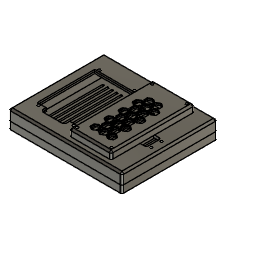
orient-beetle-screen-case-v2 v14 (Autodesk Fusion 360 design; units mm, degrees)
Autodesk Fusion 360 part; units mm, degrees
sketch "base-sketch" plane through (0, 0, 0) normal (0, 0, 1) x (1, 0, 0)
  line L0 (0, 0) -> (120, 0)
  line L1 (120, 0) -> (120, 100)
  line L2 (120, 100) -> (0, 100)
  line L3 (0, 100) -> (0, 0)
  line L4 (10, 19.5) -> (53.5, 19.5)
  line L5 (53.5, 19.5) -> (53.5, 80.5)
  line L6 (53.5, 80.5) -> (10, 80.5)
  line L7 (10, 80.5) -> (10, 19.5)
  line L8 (104, 11) -> (64, 11)
  line L9 (64, 11) -> (64, 89)
  line L10 (64, 89) -> (104, 89)
  line L11 (104, 89) -> (104, 11)
  line L12 (44.25, 86.5) -> (19.25, 86.5)
  line L13 (19.25, 86.5) -> (19.25, 80.5)
  line L14 (19.25, 80.5) -> (44.25, 80.5)
  line L15 (44.25, 80.5) -> (44.25, 86.5)
  line L16 (31.75, 19.5) -> (31.75, 80.5) construction
  line L17 (31.75, 80.5) -> (31.75, 86.5) construction
  line L18 (104, 49) -> (113.5, 49)
  line L19 (113.5, 49) -> (113.5, 65.5)
  line L20 (113.5, 65.5) -> (104, 65.5)
  line L21 (104, 65.5) -> (104, 49)
  circle A0 centre (116, 51.5) radius 1.5
  circle A1 centre (116, 63) radius 1.5
  line L22 (116, 51.5) -> (116, 63) construction
  line L23 (104, 57.25) -> (113.5, 57.25)
  circle A2 centre (12.25, 16.5) radius 1.6
  line L24 (10, 50) -> (53.5, 50) construction
  circle A3 centre (51.25, 16.5) radius 1.6
  circle A4 centre (12.25, 83.5) radius 1.6
  circle A5 centre (51.25, 83.5) radius 1.6
  line L25 (122.1, 102.1) -> (-2.1, 102.1)
  line L26 (-2.1, 102.1) -> (-2.1, -2.1)
  line L27 (-2.1, -2.1) -> (122.1, -2.1)
  line L28 (122.1, -2.1) -> (122.1, 102.1)
  point P0 (116, 57.25)
  dimension "d1" = 120
  dimension "d2" = 100
  dimension "d3" = 43.5
  dimension "d4" = 61
  dimension "d6" = 10
  dimension "d7" = 40
  dimension "d8" = 78
  dimension "d9" = 16
  dimension "d10" = 11
  dimension "d11" = 19.5
  dimension "d12" = 19.5
  dimension "d13" = 11
  dimension "d14" = 25
  dimension "d15" = 6
  dimension "d20" = 9.5
  dimension "d21" = 16.5
  dimension "d22" = 34.5
  dimension "d23" = 3
  dimension "d24" = 3
  dimension "d25" = 11.5
  dimension "d27" = 12
  dimension "d28" = 3.2
  dimension "d31" = 3.2
  dimension "d33" = 3.2
  dimension "d40" = 19.5
  dimension "d41" = 33.5
  dimension "d42" = 3.2
  dimension "d43" = 39
  dimension "d44" = 33.5
  dimension "d45" = 33.5
  dimension "d46" = 33.5
  dimension "d47" = 39
  dimension "d48" = 19.5
  dimension "d49" = 2.1
  constraint horizontal L0
  constraint vertical L1
  constraint horizontal L2
  constraint vertical L3
  constraint coincident L0.start L3.end
  constraint horizontal L4
  constraint vertical L5
  constraint horizontal L6
  constraint vertical L7
  constraint horizontal L8
  constraint vertical L9
  constraint horizontal L10
  constraint vertical L11
  constraint horizontal L12
  constraint vertical L13
  constraint horizontal L14
  constraint vertical L15
  constraint midpoint L4 L16.start
  constraint midpoint L6 L16.end
  constraint midpoint L14 L16.end
  constraint midpoint L12 L17.end
  constraint collinear L16 L17
  constraint collinear L6 L14
  constraint horizontal L18
  constraint vertical L19
  constraint horizontal L20
  constraint vertical L21
  constraint collinear L11 L21
  constraint coincident A0.centre L22.start
  constraint coincident A1.centre L22.end
  constraint parallel L19 L22
  constraint midpoint L21 L23.start
  constraint midpoint L19 L23.end
  constraint midpoint L22 P0
  constraint coincident L23 P0
  constraint midpoint L7 L24.start
  constraint midpoint L5 L24.end
  measures "d1" distance of L0.start L0.end
  measures "d2" distance of L0.start L2.end
  measures "d3" distance of L4.start L4.end
  measures "d4" distance of L4.start L6.end
  measures "d6" distance of L3 L7
  measures "d7" distance of L8.start L8.end
  measures "d8" distance of L8.start L10.end
  measures "d9" distance of L1 L11
  measures "d10" distance of L0 L8
  measures "d11" distance of L2 L6
  measures "d12" distance of L0 L4
  measures "d13" distance of L2 L10
  measures "d14" distance of L12.start L12.end
  measures "d15" distance of L12.end L13.end
  measures "d20" distance of L19.end L20.end
  measures "d21" distance of L18.end L19.end
  measures "d22" distance of L2 L20
  measures "d23" diameter of A0
  measures "d24" diameter of A1
  measures "d25" distance of A0.centre A1.centre
  measures "d27" distance of L21 A0.centre
  measures "d28" diameter of A2
  measures "d31" diameter of A3
  measures "d33" diameter of A4
  measures "d40" distance of L16 A4.centre
  measures "d41" distance of L24 A4.centre
  measures "d42" diameter of A5
  measures "d43" distance of A4.centre A5.centre
  measures "d44" distance of L24 A5.centre
  measures "d45" distance of A2.centre L24
  measures "d46" distance of L24 A3.centre
  measures "d47" distance of A2.centre A3.centre
  measures "d48" distance of L16 A2.centre
sketch "body-two-better" plane through (0, 0, 0) normal (0, 0, 1) x (1, 0, 0)
  line L0 (-14.1, 0) -> (-134.1, 0)
  line L1 (-134.1, 0) -> (-134.1, 100)
  line L2 (-134.1, 100) -> (-14.1, 100)
  line L3 (-14.1, 100) -> (-14.1, 0)
  line L4 (-2.1, 102.1) -> (-2.1, -2.1)
  line L5 (0, 0) -> (120, 0)
  line L6 (-11.6, -2.5) -> (-136.6, -2.5)
  line L7 (-136.6, -2.5) -> (-136.6, 102.5)
  line L8 (-136.6, 102.5) -> (-11.6, 102.5)
  line L9 (-11.6, 102.5) -> (-11.6, -2.5)
  line L10 (-103.1, 100) -> (-103.1, 0) construction
  line L11 (-14.1, 50) -> (-134.1, 50) construction
  line L12 (-81.35, 19.25) -> (-124.85, 19.25)
  line L13 (-124.85, 19.25) -> (-124.85, 80.75)
  line L14 (-124.85, 80.75) -> (-81.35, 80.75)
  line L15 (-81.35, 80.75) -> (-81.35, 19.25)
  line L16 (-103.1, 80.75) -> (-103.1, 19.25) construction
  line L17 (-81.35, 50) -> (-124.85, 50) construction
  circle A0 centre (-122.6, 83.5) radius 1.55
  circle A1 centre (-122.6, 16.5) radius 1.55
  line L18 (-122.6, 16.5) -> (-122.6, 26.5) construction
  line L19 (-122.6, 83.5) -> (-122.6, 73.5) construction
  circle A2 centre (-83.6, 83.5) radius 1.55
  line L20 (-83.6, 83.5) -> (-93.6, 83.5) construction
  line L21 (-122.6, 83.5) -> (-112.6, 83.5) construction
  circle A3 centre (-83.6, 16.5) radius 1.55
  line L22 (-83.6, 16.5) -> (-83.6, 26.5) construction
  line L23 (-83.6, 83.5) -> (-83.6, 73.5) construction
  line L24 (-83.6, 16.5) -> (-93.6, 16.5) construction
  line L25 (-122.6, 16.5) -> (-112.6, 16.5) construction
  line L26 (-83.6, 83.5) -> (-122.6, 16.5) construction
  line L27 (-117.1, 91.75) -> (-89.1, 91.75) construction
  line L28 (-89.1, 91.75) -> (-89.1, 80.75) construction
  line L29 (-89.1, 80.75) -> (-117.1, 80.75)
  line L30 (-117.1, 80.75) -> (-117.1, 91.75) construction
  line L31 (-117.1, 91.75) -> (-89.1, 80.75) construction
  line L32 (-89.1, 91.75) -> (-117.1, 80.75) construction
  line L33 (-53.1, 100) -> (-53.1, 0) construction
  line L34 (-73.1, 89) -> (-33.1, 89)
  line L35 (-33.1, 89) -> (-33.1, 11)
  line L36 (-33.1, 11) -> (-73.1, 11)
  line L37 (-73.1, 11) -> (-73.1, 89)
  line L38 (-73.1, 89) -> (-33.1, 11) construction
  line L39 (-33.1, 89) -> (-73.1, 11) construction
  line L40 (-33.1, 52) -> (-23.1, 52)
  line L41 (-23.1, 52) -> (-23.1, 36)
  line L42 (-23.1, 36) -> (-33.1, 36)
  line L43 (-33.1, 36) -> (-33.1, 52)
  line L44 (-33.1, 52) -> (-23.1, 36) construction
  line L45 (-23.1, 52) -> (-33.1, 36) construction
  circle A4 centre (-20.1, 49.75) radius 1.3
  circle A5 centre (-20.1, 38.25) radius 1.3
  line L46 (-20.1, 38.25) -> (-20.1, 42.25) construction
  line L47 (-20.1, 49.75) -> (-20.1, 45.75) construction
  line L48 (-20.1, 49.75) -> (-20.1, 38.25) construction
  line L49 (-23.1, 44) -> (-20.1, 44) construction
  circle A6 centre (-34.1, 91.5) radius 1.4
  circle A7 centre (-34.1, 8.5) radius 1.4
  circle A8 centre (-72.1, 8.5) radius 1.4
  circle A9 centre (-72.1, 91.5) radius 1.4
  line L50 (-34.1, 91.5) -> (-36.1, 91.5) construction
  line L51 (-34.1, 8.5) -> (-36.1, 8.5) construction
  line L52 (-34.1, 8.5) -> (-34.1, 10.5) construction
  line L53 (-72.1, 8.5) -> (-72.1, 10.5) construction
  line L54 (-72.1, 8.5) -> (-70.1, 8.5) construction
  line L55 (-72.1, 91.5) -> (-72.1, 89.5) construction
  line L56 (-72.1, 91.5) -> (-70.1, 91.5) construction
  line L57 (-34.1, 91.5) -> (-34.1, 89.5) construction
  line L58 (-34.1, 91.5) -> (-72.1, 8.5) construction
  line L59 (-115.1, 19.25) -> (-91.1, 19.25)
  line L60 (-91.1, 19.25) -> (-91.1, 13.25)
  line L61 (-91.1, 13.25) -> (-115.1, 13.25)
  line L62 (-115.1, 13.25) -> (-115.1, 19.25)
  line L63 (-115.1, 19.25) -> (-91.1, 13.25) construction
  line L64 (-91.1, 19.25) -> (-115.1, 13.25) construction
  line L65 (-28.1, 94) -> (-28.1, 6) construction
  line L66 (-28.1, 6) -> (-78.1, 6) construction
  line L67 (-78.1, 6) -> (-78.1, 94) construction
  line L68 (-78.1, 94) -> (-28.1, 94) construction
  point P0 (-103.1, 50)
  point P1 (-103.1, 50)
  point P2 (-103.1, 50)
  point P3 (-103.1, 80.75)
  point P4 (-103.1, 86.25)
  point P5 (-103.1, 80.75)
  point P6 (-53.1, 50)
  point P7 (-53.1, 50)
  point P8 (-28.1, 44)
  point P9 (-33.1, 44)
  point P10 (-33.1, 44)
  point P11 (-53.1, 50)
  point P12 (-103.1, 19.25)
  point P13 (-103.1, 16.25)
  point P14 (-103.1, 19.25)
  dimension "d150" = 120
  dimension "d151" = 100
  dimension "d152" = 12
  dimension "d153" = -2.5
  dimension "d154" = 31
  dimension "d155" = 43.5
  dimension "d156" = 61.5
  dimension "d157" = 3.1
  dimension "d158" = 3.1
  dimension "d159" = 10
  dimension "d160" = 10
  dimension "d162" = 3.1
  dimension "d163" = 10
  dimension "d164" = 39
  dimension "d165" = 67
  dimension "d166" = 3.1
  dimension "d167" = 10
  dimension "d168" = 10
  dimension "d169" = 10
  dimension "d170" = 10
  dimension "d171" = 10
  dimension "d174" = 28
  dimension "d175" = 11
  dimension "d176" = 50
  dimension "d177" = 40
  dimension "d178" = 78
  dimension "d179" = 16
  dimension "d180" = 10
  dimension "d184" = 2.6
  dimension "d185" = 2.6
  dimension "d186" = 4
  dimension "d187" = 4
  dimension "d188" = 11.5
  dimension "d190" = 3
  dimension "d198" = 2.8
  dimension "d199" = 2.8
  dimension "d200" = 2.8
  dimension "d201" = 2.8
  dimension "d206" = 2
  dimension "d207" = 2
  dimension "d208" = 2
  dimension "d209" = 2
  dimension "d210" = 2
  dimension "d211" = 2
  dimension "d212" = 2
  dimension "d213" = 2
  dimension "d214" = 83
  dimension "d215" = 38
  dimension "d224" = 44
  dimension "d225" = 6
  dimension "d227" = 24
  dimension "d247" = -5
  constraint horizontal L0
  constraint vertical L1
  constraint horizontal L2
  constraint vertical L3
  constraint collinear L0 L5
  constraint coincident L2 L10.start
  constraint coincident L0 L10.end
  constraint perpendicular L0 L10
  constraint midpoint L3 L11.start
  constraint midpoint L1 L11.end
  constraint horizontal L12
  constraint vertical L13
  constraint horizontal L14
  constraint vertical L15
  constraint midpoint L10 P2
  constraint midpoint L14 P5
  constraint midpoint L12 P14
  constraint midpoint L15 L17.start
  constraint midpoint L13 L17.end
  constraint midpoint L17 P2
  constraint coincident A1.centre L18.start
  constraint vertical L18
  constraint coincident A0.centre L19.start
  constraint vertical L19
  constraint collinear L18 L19
  constraint coincident A2.centre L20.start
  constraint horizontal L20
  constraint perpendicular L19 L21
  constraint collinear L20 L21
  constraint coincident A3.centre L22.start
  constraint vertical L22
  constraint perpendicular L20 L23
  constraint collinear L22 L23
  constraint perpendicular L22 L24
  constraint perpendicular L18 L25
  constraint collinear L24 L25
  constraint midpoint L26 P2
  constraint midpoint L16 P2
  constraint coincident P5 P3
  constraint horizontal L27
  constraint perpendicular L27 L28
  constraint parallel L27 L29
  constraint parallel L28 L30
  constraint coincident L31 P4
  constraint coincident L32 P4
  constraint midpoint L29 P5
  constraint vertical L33
  constraint coincident L2 L33.start
  constraint coincident L0 L33.end
  constraint midpoint L33 P11
  constraint horizontal L34
  constraint perpendicular L34 L35
  constraint parallel L34 L36
  constraint parallel L35 L37
  constraint coincident L38 P11
  constraint coincident L39 P11
  constraint coincident P11 P7
  constraint horizontal L40
  constraint perpendicular L40 L41
  constraint parallel L40 L42
  constraint parallel L41 L43
  constraint coincident L44 P8
  constraint coincident L45 P8
  constraint coincident A5.centre L46.start
  constraint vertical L46
  constraint coincident A4.centre L47.start
  constraint vertical L47
  constraint collinear L46 L47
  constraint midpoint L41 L49.start
  constraint perpendicular L41 L49
  constraint midpoint L48 L49.end
  constraint coincident L35 P10
  constraint midpoint L43 P10
  constraint coincident P10 P9
  constraint coincident A6.centre L50.start
  constraint horizontal L50
  constraint coincident A7.centre L51.start
  constraint horizontal L51
  constraint perpendicular L51 L52
  constraint coincident A8.centre L53.start
  constraint vertical L53
  constraint perpendicular L53 L54
  constraint coincident A9.centre L55.start
  constraint vertical L55
  constraint perpendicular L55 L56
  constraint vertical L57
  constraint collinear L50 L56
  constraint collinear L53 L55
  constraint collinear L51 L54
  constraint collinear L52 L57
  constraint midpoint L58 P11
  constraint coincident P14 P12
  constraint horizontal L59
  constraint perpendicular L59 L60
  constraint parallel L59 L61
  constraint parallel L60 L62
  constraint coincident L63 P13
  constraint coincident L64 P13
  constraint midpoint L59 P14
  measures "d150" distance of L0.start L0.end
  measures "d151" distance of L0.start L2.end
  measures "d152" distance of L3 L4
  measures "d154" distance of L1 L10
  measures "d155" distance of L12.start L12.end
  measures "d156" distance of L12.start L14.end
  measures "d157" diameter of A0
  measures "d158" diameter of A1
  measures "d159" distance of A0.centre L19.end
  measures "d160" distance of A1.centre L18.end
  measures "d162" diameter of A2
  measures "d163" distance of A2.centre L20.end
  measures "d164" distance of A0.centre A2.centre
  measures "d165" distance of A0.centre A1.centre
  measures "d166" diameter of A3
  measures "d167" distance of A3.centre L22.end
  measures "d168" distance of A2.centre L23.end
  measures "d169" distance of A3.centre L24.end
  measures "d170" distance of A1.centre L25.end
  measures "d171" distance of A0.centre L21.end
  measures "d174" distance of L28.end L29.end
  measures "d175" distance of L27.end L28.end
  measures "d176" distance of L10 L33
  measures "d177" distance of L35.end L36.end
  measures "d178" distance of L34.start L36.end
  measures "d179" distance of L40.end L41.end
  measures "d180" distance of L40.start L40.end
  measures "d184" diameter of A4
  measures "d185" diameter of A5
  measures "d186" distance of A5.centre L46.end
  measures "d187" distance of A4.centre L47.end
  measures "d188" distance of A4.centre A5.centre
  measures "d190" distance of L49.start L49.end
  measures "d198" diameter of A6
  measures "d199" diameter of A7
  measures "d200" diameter of A8
  measures "d201" diameter of A9
  measures "d206" distance of A7.centre L51.end
  measures "d207" distance of A7.centre L52.end
  measures "d208" distance of A8.centre L53.end
  measures "d209" distance of A8.centre L54.end
  measures "d210" distance of A9.centre L55.end
  measures "d211" distance of A9.centre L56.end
  measures "d212" distance of A6.centre L57.end
  measures "d213" distance of A6.centre L50.end
  measures "d214" distance of A6.centre A7.centre
  measures "d215" distance of A7.centre A8.centre
  measures "d224" distance of L0 P8
  measures "d225" distance of L59.start L61.end
  measures "d227" distance of L60.end L61.end
extrude "wall-extrude" add sketch "body-two-better" against normal blind 10 contours L6 L7 L8 L9 makes body 1
extrude "face-extrude" add sketch "body-two-better" against normal blind 3 contours L0 L1 L2 L3 bodies 1
sketch "expansion-sketch" plane through (0, 0, 0) normal (0, 0, 1) x (1, 0, 0)
  line L0 (-78.1, 6) -> (-78.1, 94)
  line L1 (-78.1, 94) -> (-28.1, 94)
  line L2 (-28.1, 6) -> (-78.1, 6)
  line L3 (-28.1, 94) -> (-28.1, 6)
  line L4 (-53.1, 94) -> (-53.1, 6) construction
  line L5 (-78.1, 50) -> (-28.1, 50) construction
  line L6 (-53.1, 54) -> (-56.5641, 52)
  line L7 (-56.5641, 52) -> (-56.5641, 48)
  line L8 (-56.5641, 48) -> (-53.1, 46)
  line L9 (-53.1, 46) -> (-49.6359, 48)
  line L10 (-49.6359, 48) -> (-49.6359, 52)
  line L11 (-49.6359, 52) -> (-53.1, 54)
  line L12 (-44.1, 46) -> (-40.6359, 48)
  line L13 (-40.6359, 48) -> (-40.6359, 52)
  line L14 (-40.6359, 52) -> (-44.1, 54)
  line L15 (-44.1, 54) -> (-47.5641, 52)
  line L16 (-47.5641, 48) -> (-44.1, 46)
  line L17 (-47.5641, 52) -> (-47.5641, 48)
  line L18 (-62.1, 46) -> (-58.6359, 48)
  line L19 (-58.6359, 48) -> (-58.6359, 52)
  line L20 (-58.6359, 52) -> (-62.1, 54)
  line L21 (-62.1, 54) -> (-65.5641, 52)
  line L22 (-65.5641, 48) -> (-62.1, 46)
  line L23 (-65.5641, 52) -> (-65.5641, 48)
  line L24 (-53.1, 50) -> (-54.8321, 53) construction
  line L25 (-53.1, 50) -> (-51.3679, 53) construction
  line L26 (-48.6, 61.7942) -> (-52.0641, 59.7942)
  line L27 (-52.0641, 59.7942) -> (-52.0641, 55.7942)
  line L28 (-52.0641, 55.7942) -> (-48.6, 53.7942)
  line L29 (-48.6, 53.7942) -> (-45.1359, 55.7942)
  line L30 (-45.1359, 59.7942) -> (-48.6, 61.7942)
  line L31 (-45.1359, 55.7942) -> (-45.1359, 59.7942)
  line L32 (-57.6, 61.7942) -> (-61.0641, 59.7942)
  line L33 (-61.0641, 59.7942) -> (-61.0641, 55.7942)
  line L34 (-61.0641, 55.7942) -> (-57.6, 53.7942)
  line L35 (-57.6, 53.7942) -> (-54.1359, 55.7942)
  line L36 (-54.1359, 59.7942) -> (-57.6, 61.7942)
  line L37 (-54.1359, 55.7942) -> (-54.1359, 59.7942)
  line L38 (-62.1, 69.5) -> (-65.5641, 67.5)
  line L39 (-65.5641, 67.5) -> (-65.5641, 63.5)
  line L40 (-65.5641, 63.5) -> (-62.1, 61.5)
  line L41 (-62.1, 61.5) -> (-58.6359, 63.5)
  line L42 (-58.6359, 67.5) -> (-62.1, 69.5)
  line L43 (-58.6359, 63.5) -> (-58.6359, 67.5)
  line L44 (-54.1359, 75.2942) -> (-57.6, 77.2942)
  line L45 (-57.6, 77.2942) -> (-61.0641, 75.2942)
  line L46 (-61.0641, 75.2942) -> (-61.0641, 71.2942)
  line L47 (-61.0641, 71.2942) -> (-57.6, 69.2942)
  line L48 (-54.1359, 71.2942) -> (-54.1359, 75.2942)
  line L49 (-57.6, 69.2942) -> (-54.1359, 71.2942)
  line L50 (-48.6, 69.2942) -> (-45.1359, 71.2942)
  line L51 (-45.1359, 71.2942) -> (-45.1359, 75.2942)
  line L52 (-45.1359, 75.2942) -> (-48.6, 77.2942)
  line L53 (-48.6, 77.2942) -> (-52.0641, 75.2942)
  line L54 (-52.0641, 71.2942) -> (-48.6, 69.2942)
  line L55 (-52.0641, 75.2942) -> (-52.0641, 71.2942)
  line L56 (-53.1, 69.5) -> (-56.5641, 67.5)
  line L57 (-56.5641, 67.5) -> (-56.5641, 63.5)
  line L58 (-56.5641, 63.5) -> (-53.1, 61.5)
  line L59 (-53.1, 61.5) -> (-49.6359, 63.5)
  line L60 (-49.6359, 67.5) -> (-53.1, 69.5)
  line L61 (-49.6359, 63.5) -> (-49.6359, 67.5)
  line L62 (-40.6359, 67.5) -> (-44.1, 69.5)
  line L63 (-44.1, 69.5) -> (-47.5641, 67.5)
  line L64 (-47.5641, 67.5) -> (-47.5641, 63.5)
  line L65 (-47.5641, 63.5) -> (-44.1, 61.5)
  line L66 (-40.6359, 63.5) -> (-40.6359, 67.5)
  line L67 (-44.1, 61.5) -> (-40.6359, 63.5)
  line L68 (-62.1, 38.5) -> (-65.5641, 36.5)
  line L69 (-65.5641, 36.5) -> (-65.5641, 32.5)
  line L70 (-65.5641, 32.5) -> (-62.1, 30.5)
  line L71 (-62.1, 30.5) -> (-58.6359, 32.5)
  line L72 (-58.6359, 36.5) -> (-62.1, 38.5)
  line L73 (-58.6359, 32.5) -> (-58.6359, 36.5)
  line L74 (-54.1359, 44.2942) -> (-57.6, 46.2942)
  line L75 (-57.6, 46.2942) -> (-61.0641, 44.2942)
  line L76 (-61.0641, 44.2942) -> (-61.0641, 40.2942)
  line L77 (-61.0641, 40.2942) -> (-57.6, 38.2942)
  line L78 (-54.1359, 40.2942) -> (-54.1359, 44.2942)
  line L79 (-57.6, 38.2942) -> (-54.1359, 40.2942)
  line L80 (-48.6, 38.2942) -> (-45.1359, 40.2942)
  line L81 (-45.1359, 40.2942) -> (-45.1359, 44.2942)
  line L82 (-45.1359, 44.2942) -> (-48.6, 46.2942)
  line L83 (-48.6, 46.2942) -> (-52.0641, 44.2942)
  line L84 (-52.0641, 40.2942) -> (-48.6, 38.2942)
  line L85 (-52.0641, 44.2942) -> (-52.0641, 40.2942)
  line L86 (-53.1, 38.5) -> (-56.5641, 36.5)
  line L87 (-56.5641, 36.5) -> (-56.5641, 32.5)
  line L88 (-56.5641, 32.5) -> (-53.1, 30.5)
  line L89 (-53.1, 30.5) -> (-49.6359, 32.5)
  line L90 (-49.6359, 36.5) -> (-53.1, 38.5)
  line L91 (-49.6359, 32.5) -> (-49.6359, 36.5)
  line L92 (-40.6359, 36.5) -> (-44.1, 38.5)
  line L93 (-44.1, 38.5) -> (-47.5641, 36.5)
  line L94 (-47.5641, 36.5) -> (-47.5641, 32.5)
  line L95 (-47.5641, 32.5) -> (-44.1, 30.5)
  line L96 (-40.6359, 32.5) -> (-40.6359, 36.5)
  line L97 (-44.1, 30.5) -> (-40.6359, 32.5)
  line L98 (-62.1, 23) -> (-65.5641, 21)
  line L99 (-65.5641, 21) -> (-65.5641, 17)
  line L100 (-65.5641, 17) -> (-62.1, 15)
  line L101 (-62.1, 15) -> (-58.6359, 17)
  line L102 (-58.6359, 21) -> (-62.1, 23)
  line L103 (-58.6359, 17) -> (-58.6359, 21)
  line L104 (-54.1359, 28.7942) -> (-57.6, 30.7942)
  line L105 (-57.6, 30.7942) -> (-61.0641, 28.7942)
  line L106 (-61.0641, 28.7942) -> (-61.0641, 24.7942)
  line L107 (-61.0641, 24.7942) -> (-57.6, 22.7942)
  line L108 (-54.1359, 24.7942) -> (-54.1359, 28.7942)
  line L109 (-57.6, 22.7942) -> (-54.1359, 24.7942)
  line L110 (-48.6, 22.7942) -> (-45.1359, 24.7942)
  line L111 (-45.1359, 24.7942) -> (-45.1359, 28.7942)
  line L112 (-45.1359, 28.7942) -> (-48.6, 30.7942)
  line L113 (-48.6, 30.7942) -> (-52.0641, 28.7942)
  line L114 (-52.0641, 24.7942) -> (-48.6, 22.7942)
  line L115 (-52.0641, 28.7942) -> (-52.0641, 24.7942)
  line L116 (-53.1, 23) -> (-56.5641, 21)
  line L117 (-56.5641, 21) -> (-56.5641, 17)
  line L118 (-56.5641, 17) -> (-53.1, 15)
  line L119 (-53.1, 15) -> (-49.6359, 17)
  line L120 (-49.6359, 21) -> (-53.1, 23)
  line L121 (-49.6359, 17) -> (-49.6359, 21)
  line L122 (-40.6359, 21) -> (-44.1, 23)
  line L123 (-44.1, 23) -> (-47.5641, 21)
  line L124 (-47.5641, 21) -> (-47.5641, 17)
  line L125 (-47.5641, 17) -> (-44.1, 15)
  line L126 (-40.6359, 17) -> (-40.6359, 21)
  line L127 (-44.1, 15) -> (-40.6359, 17)
  point P0 (-53.1, 50)
  point P1 (-53.1, 50)
  dimension "d266" = 4
  dimension "d267" = 60
  dimension "d270" = 9
  dimension "d271" = 0
  dimension "d278" = 9
  dimension "d279" = 9
  dimension "d282" = 15.5
  dimension "d283" = 0
  constraint midpoint L1 L4.start
  constraint midpoint L2 L4.end
  constraint midpoint L0 L5.start
  constraint midpoint L3 L5.end
  constraint midpoint L5 P1
  constraint coincident P1 P0
  constraint midpoint L6 L24.end
  constraint midpoint L11 L25.end
  measures "d266" distance of L6.start P1
  measures "d267" angle of L3 L11
extrude "expansion-extrude" add sketch "expansion-sketch" along normal blind 8 separate body makes body 2
extrude "expansion-extrude-cut" cut sketch "body-two-better" along normal blind 6 contours L34 L35 L36 L37 L43 bodies 1 2
extrude "Extrude20" cut sketch "body-two-better" along normal blind 20 contours A6 | A7 | A8 | A9 bodies 2
move_face "OffsetFaces5" offset -2 2 faces at (-78.1, 35.3333, 2.6667) (-28.1, 64.6667, 2.6667) on bodies 2
move_face "OffsetFaces6" offset 2 2 faces at (-45.4333, 6, 2.6667) (-60.7667, 94, 2.6667) on bodies 2
sketch "cable-cut" plane through (0, 102.5, 0) normal (0, 1, 0) x (-1, 0, 0)
  line L0 (136.6, 0) -> (11.6, 0)
  line L1 (11.6, -10) -> (136.6, -10)
  line L2 (65.1, 6) -> (41.1, 6)
  line L3 (41.1, 6) -> (41.1, -7)
  line L4 (41.1, -7) -> (65.1, -7)
  line L5 (65.1, -7) -> (65.1, 6)
  line L6 (65.1, 6) -> (41.1, -7) construction
  line L7 (41.1, 6) -> (65.1, -7) construction
  line L8 (76.1, 4) -> (30.1, 4) construction
  line L9 (65.1, 4) -> (41.1, 4) construction
  line L10 (11.6, 0) -> (11.6, -10)
  line L11 (136.6, -10) -> (136.6, 0)
  line L12 (76.1, 0) -> (76.1, 8)
  line L13 (30.1, 0) -> (30.1, 8)
  point P0 (53.1, -0.5)
  point P1 (53.1, 4)
  point P2 (53.1, 4)
  dimension "d294" = 24
  dimension "d295" = 13
  dimension "d296" = 2
  constraint horizontal L2
  constraint perpendicular L2 L3
  constraint parallel L2 L4
  constraint parallel L3 L5
  constraint coincident L6 P0
  constraint coincident L7 P0
  constraint midpoint L8 P2
  constraint coincident L5 L9.start
  constraint coincident L3 L9.end
  constraint perpendicular L3 L9
  constraint midpoint L9 P2
  constraint coincident P2 P1
  constraint midpoint L8.start L12
  constraint midpoint L8.end L13
  measures "d294" distance of L3.end L4.end
  measures "d295" distance of L2.end L3.end
  measures "d296" distance of L2 L9
extrude "Extrude21" cut sketch "cable-cut" against normal blind 39 contours L0 L3 L4 L5 bodies 1
extrude "Extrude22" cut sketch "cable-cut" against normal blind 40 contours L0 L2 L3 L5 bodies 2
extrude "Extrude23" add 1 faces at (-54.1, -1.6667, -10) along direction (0, 0, -1) blind 10 on bodies 1 bodies 1
sketch "bottom-sketch" plane through (0, 0, -20) normal (0, 0, -1) x (1, 0, 0)
  line L0 (-14.1, -100) -> (-134.1, -100)
  line L1 (-134.1, -100) -> (-134.1, 0)
  line L2 (-134.1, 0) -> (-14.1, 0)
  line L3 (-14.1, 0) -> (-14.1, -100)
  line L4 (-136.6, -102.5) -> (-11.6, -102.5)
  line L5 (-11.6, -102.5) -> (-11.6, 2.5)
  line L6 (-11.6, 2.5) -> (-136.6, 2.5)
  line L7 (-136.6, 2.5) -> (-136.6, -102.5)
  line L8 (-14.1, 0) -> (-134.1, 0)
  line L9 (-14.1, -100) -> (-14.1, 0)
  line L10 (-134.1, -100) -> (-14.1, -100)
  line L11 (-134.1, 0) -> (-134.1, -100)
extrude "Extrude24" add sketch "bottom-sketch" against normal blind 2 contours L0 L1 L2 L3 L8 L9 L10 L11 bodies 1
ref_plane "WorkPlane1" through (0, 0, -12) normal (0, 0, 1) x (1, 0, 0)
split "Split1" by plane through (0, 0, -12) normal (0, 0, 1) bodies 1 makes body 3 at (-21.4463, 80.8218, 0)
sketch "inner-sketch" plane through (0, 0, -18) normal (0, 0, 1) x (-1, 0, 0)
  line L0 (134.1, -100) -> (134.1, 0)
  line L1 (134.1, 0) -> (14.1, 0)
  line L2 (14.1, 0) -> (14.1, -100)
  line L3 (14.1, -100) -> (134.1, -100)
  line L4 (132.1, -98) -> (132.1, -2)
  line L5 (132.1, -2) -> (16.1, -2)
  line L6 (16.1, -2) -> (16.1, -98)
  line L7 (16.1, -98) -> (132.1, -98)
  dimension "d312" = -2
extrude "Extrude25" add sketch "inner-sketch" along normal blind 8 bodies 1
fillet "Fillet29" radius 2 8 edges at (-76.1, 4, 4) (-30.1, 4, 4) (-33.1, 89, 3) (-30.1, 96, 4) (-73.1, 89, 3) (-76.1, 96, 4) (-73.1, 11, 3) (-33.1, 11, 3) on bodies 2
fillet "Fillet30" radius 2 2 edges at (-41.1, 92.5, 6) (-65.1, 92.5, 6) on bodies 2
fillet "Fillet32" radius 2 23 edges at (-11.6, -2.5, -6) (-136.6, -2.5, -6) (-136.6, 102.5, -6) (-11.6, 102.5, -6) (-14.1, 100, -7.5) (-14.1, 0, -7.5) (-134.1, 0, -7.5) (-134.1, 100, -7.5) (-65.1, 89, -1.5) (-41.1, 89, -1.5) (-23.1, 36, -1.5) (-33.1, 36, -1.5) (-33.1, 52, -1.5) (-33.1, 11, -1.5) (-73.1, 11, -1.5) (-73.1, 89, -1.5) (-23.1, 52, -1.5) (-65.1, 101.25, -7) (-41.1, 101.25, -7) (-91.1, 13.25, -1.5) (-115.1, 13.25, -1.5) (-115.1, 19.25, -1.5) (-91.1, 19.25, -1.5) on bodies 3
chamfer "Chamfer1" distance 1 angle 45 12 edges at (-124.85, 50, 0) (-103.1, 80.75, 0) (-81.35, 50, 0) (-85.225, 19.25, 0) (-90.5142, 18.6642, 0) (-91.1, 16.25, 0) (-91.6858, 13.8358, 0) (-103.1, 13.25, 0) (-114.5142, 13.8358, 0) (-115.1, 16.25, 0) (-115.6858, 18.6642, 0) (-120.975, 19.25, 0) on bodies 3
chamfer "Chamfer2" distance 2 angle 45 9 edges at (-136.6, 50, 0) (-136.0142, -1.9142, 0) (-74.1, -2.5, 0) (-12.1858, -1.9142, 0) (-11.6, 50, 0) (-12.1858, 101.9142, 0) (-27.35, 102.5, 0) (-99.85, 102.5, 0) (-136.0142, 101.9142, 0) on bodies 3
chamfer "Chamfer3" distance 2 angle 45 8 edges at (-53.1, 96, 8) (-75.5142, 95.4142, 8) (-76.1, 50, 8) (-75.5142, 4.5858, 8) (-53.1, 4, 8) (-30.6858, 4.5858, 8) (-30.1, 50, 8) (-30.6858, 95.4142, 8) on bodies 2
chamfer "Chamfer4" distance 0.5 angle 45 120 edges at (-47.5641, 34.5, 8) (-45.8321, 31.5, 8) (-42.3679, 31.5, 8) (-42.3679, 37.5, 8) (-45.8321, 37.5, 8) (-40.6359, 34.5, 8) (-49.6359, 34.5, 8) (-51.3679, 31.5, 8) (-54.8321, 31.5, 8) (-56.5641, 34.5, 8) (-54.8321, 37.5, 8) (-51.3679, 37.5, 8) (-60.3679, 37.5, 8) (-63.8321, 37.5, 8) (-65.5641, 34.5, 8) (-63.8321, 31.5, 8) (-60.3679, 31.5, 8) (-58.6359, 34.5, 8) (-61.0641, 26.7942, 8) (-59.3321, 29.7942, 8) (-55.8679, 29.7942, 8) (-54.1359, 26.7942, 8) (-55.8679, 23.7942, 8) (-59.3321, 23.7942, 8) (-52.0641, 26.7942, 8) (-50.3321, 29.7942, 8) (-46.8679, 29.7942, 8) (-45.1359, 26.7942, 8) (-46.8679, 23.7942, 8) (-50.3321, 23.7942, 8) (-51.3679, 22, 8) (-54.8321, 22, 8) (-56.5641, 19, 8) (-54.8321, 16, 8) (-51.3679, 16, 8) (-49.6359, 19, 8) (-47.5641, 19, 8) (-45.8321, 16, 8) (-42.3679, 16, 8) (-40.6359, 19, 8) (-42.3679, 22, 8) (-45.8321, 22, 8) (-58.6359, 19, 8) (-60.3679, 16, 8) (-63.8321, 16, 8) (-65.5641, 19, 8) (-63.8321, 22, 8) (-60.3679, 22, 8) (-61.0641, 42.2942, 8) (-59.3321, 39.2942, 8) (-55.8679, 39.2942, 8) (-54.1359, 42.2942, 8) (-55.8679, 45.2942, 8) (-59.3321, 45.2942, 8) (-52.0641, 42.2942, 8) (-50.3321, 39.2942, 8) (-46.8679, 39.2942, 8) (-45.1359, 42.2942, 8) (-46.8679, 45.2942, 8) (-50.3321, 45.2942, 8) (-61.0641, 57.7942, 8) (-59.3321, 54.7942, 8) (-55.8679, 54.7942, 8) (-54.1359, 57.7942, 8) (-59.3321, 60.7942, 8) (-55.8679, 60.7942, 8) (-65.5641, 50, 8) (-63.8321, 47, 8) (-60.3679, 47, 8) (-63.8321, 53, 8) (-60.3679, 53, 8) (-58.6359, 50, 8) (-56.5641, 50, 8) (-54.8321, 47, 8) (-51.3679, 47, 8) (-49.6359, 50, 8) (-51.3679, 53, 8) (-54.8321, 53, 8) (-45.8321, 53, 8) (-47.5641, 50, 8) (-45.8321, 47, 8) (-42.3679, 47, 8) (-40.6359, 50, 8) (-42.3679, 53, 8) (-46.8679, 54.7942, 8) (-50.3321, 54.7942, 8) (-52.0641, 57.7942, 8) (-50.3321, 60.7942, 8) (-46.8679, 60.7942, 8) (-45.1359, 57.7942, 8) (-40.6359, 65.5, 8) (-42.3679, 68.5, 8) (-45.8321, 68.5, 8) (-47.5641, 65.5, 8) (-45.8321, 62.5, 8) (-42.3679, 62.5, 8) (-51.3679, 62.5, 8) (-58.6359, 65.5, 8) (-54.8321, 62.5, 8) (-56.5641, 65.5, 8) (-54.8321, 68.5, 8) (-51.3679, 68.5, 8) (-49.6359, 65.5, 8) (-60.3679, 68.5, 8) (-63.8321, 68.5, 8) (-65.5641, 65.5, 8) (-63.8321, 62.5, 8) (-60.3679, 62.5, 8) (-59.3321, 70.2942, 8) (-61.0641, 73.2942, 8) (-59.3321, 76.2942, 8) (-55.8679, 76.2942, 8) (-54.1359, 73.2942, 8) (-55.8679, 70.2942, 8) (-52.0641, 73.2942, 8) (-50.3321, 76.2942, 8) (-46.8679, 76.2942, 8) (-45.1359, 73.2942, 8) (-46.8679, 70.2942, 8) (-50.3321, 70.2942, 8) on bodies 2
move_face "OffsetFaces7" offset -0.5 4 faces at (-14.1, 33.3333, -11.3333) (-54.1, 0, -10.6667) (-134.1, 66.6667, -11.3333) (-54.1, 100, -11.3333) on bodies 1
fillet "Fillet33" radius 2 12 edges at (-11.6, 102.5, -16) (-14.6, 99.5, -11) (-11.6, -2.5, -16) (-14.6, 0.5, -11) (-136.6, -2.5, -16) (-133.6, 0.5, -11) (-136.6, 102.5, -16) (-133.6, 99.5, -11) (-16.1, 98, -14) (-132.1, 98, -14) (-132.1, 2, -14) (-16.1, 2, -14) on bodies 1
sketch "bottom-cut-sketch" plane through (0, 0, -20) normal (0, 0, -1) x (1, 0, 0)
  arc A0 (-136.6, -100.5) -> (-134.6, -102.5) centre (-134.6, -100.5) ccw
  line L0 (-134.6, -102.5) -> (-13.6, -102.5)
  arc A1 (-13.6, -102.5) -> (-11.6, -100.5) centre (-13.6, -100.5) ccw
  line L1 (-11.6, -100.5) -> (-11.6, 0.5)
  arc A2 (-11.6, 0.5) -> (-13.6, 2.5) centre (-13.6, 0.5) ccw
  line L2 (-13.6, 2.5) -> (-134.6, 2.5)
  arc A3 (-134.6, 2.5) -> (-136.6, 0.5) centre (-134.6, 0.5) ccw
  line L3 (-136.6, 0.5) -> (-136.6, -100.5)
  line L4 (-132.1, -98) -> (-132.1, -2)
  line L5 (-132.1, -2) -> (-16.1, -2)
  line L6 (-16.1, -2) -> (-16.1, -98)
  line L7 (-16.1, -98) -> (-132.1, -98)
  line L8 (-74.1, -2) -> (-74.1, -98) construction
  line L9 (-73.1, -10) -> (-75.1, -10)
  line L10 (-75.1, -10) -> (-75.1, -90)
  line L11 (-75.1, -90) -> (-73.1, -90)
  line L12 (-73.1, -90) -> (-73.1, -10)
  line L13 (-73.1, -10) -> (-75.1, -90) construction
  line L14 (-75.1, -10) -> (-73.1, -90) construction
  line L15 (-30.1, -10) -> (-30.1, -90)
  line L16 (-30.1, -90) -> (-28.1, -90)
  line L17 (-28.1, -10) -> (-30.1, -10)
  line L18 (-28.1, -90) -> (-28.1, -10)
  line L19 (-35.1, -10) -> (-35.1, -90)
  line L20 (-35.1, -90) -> (-33.1, -90)
  line L21 (-33.1, -10) -> (-35.1, -10)
  line L22 (-33.1, -90) -> (-33.1, -10)
  line L23 (-40.1, -10) -> (-40.1, -90)
  line L24 (-40.1, -90) -> (-38.1, -90)
  line L25 (-38.1, -10) -> (-40.1, -10)
  line L26 (-38.1, -90) -> (-38.1, -10)
  line L27 (-45.1, -10) -> (-45.1, -90)
  line L28 (-45.1, -90) -> (-43.1, -90)
  line L29 (-43.1, -10) -> (-45.1, -10)
  line L30 (-43.1, -90) -> (-43.1, -10)
  line L31 (-50.1, -10) -> (-50.1, -90)
  line L32 (-50.1, -90) -> (-48.1, -90)
  line L33 (-48.1, -10) -> (-50.1, -10)
  line L34 (-48.1, -90) -> (-48.1, -10)
  line L35 (-55.1, -10) -> (-55.1, -90)
  line L36 (-55.1, -90) -> (-53.1, -90)
  line L37 (-53.1, -10) -> (-55.1, -10)
  line L38 (-53.1, -90) -> (-53.1, -10)
  line L39 (-60.1, -10) -> (-60.1, -90)
  line L40 (-60.1, -90) -> (-58.1, -90)
  line L41 (-58.1, -10) -> (-60.1, -10)
  line L42 (-58.1, -90) -> (-58.1, -10)
  line L43 (-65.1, -10) -> (-65.1, -90)
  line L44 (-65.1, -90) -> (-63.1, -90)
  line L45 (-63.1, -10) -> (-65.1, -10)
  line L46 (-63.1, -90) -> (-63.1, -10)
  line L47 (-70.1, -10) -> (-70.1, -90)
  line L48 (-70.1, -90) -> (-68.1, -90)
  line L49 (-68.1, -10) -> (-70.1, -10)
  line L50 (-68.1, -90) -> (-68.1, -10)
  line L51 (-80.1, -10) -> (-80.1, -90)
  line L52 (-80.1, -90) -> (-78.1, -90)
  line L53 (-78.1, -10) -> (-80.1, -10)
  line L54 (-78.1, -90) -> (-78.1, -10)
  line L55 (-85.1, -10) -> (-85.1, -90)
  line L56 (-85.1, -90) -> (-83.1, -90)
  line L57 (-83.1, -10) -> (-85.1, -10)
  line L58 (-83.1, -90) -> (-83.1, -10)
  line L59 (-90.1, -10) -> (-90.1, -90)
  line L60 (-90.1, -90) -> (-88.1, -90)
  line L61 (-88.1, -10) -> (-90.1, -10)
  line L62 (-88.1, -90) -> (-88.1, -10)
  line L63 (-95.1, -10) -> (-95.1, -90)
  line L64 (-95.1, -90) -> (-93.1, -90)
  line L65 (-93.1, -10) -> (-95.1, -10)
  line L66 (-93.1, -90) -> (-93.1, -10)
  line L67 (-100.1, -10) -> (-100.1, -90)
  line L68 (-100.1, -90) -> (-98.1, -90)
  line L69 (-98.1, -10) -> (-100.1, -10)
  line L70 (-98.1, -90) -> (-98.1, -10)
  line L71 (-105.1, -10) -> (-105.1, -90)
  line L72 (-105.1, -90) -> (-103.1, -90)
  line L73 (-103.1, -10) -> (-105.1, -10)
  line L74 (-103.1, -90) -> (-103.1, -10)
  line L75 (-110.1, -10) -> (-110.1, -90)
  line L76 (-110.1, -90) -> (-108.1, -90)
  line L77 (-108.1, -10) -> (-110.1, -10)
  line L78 (-108.1, -90) -> (-108.1, -10)
  line L79 (-115.1, -10) -> (-115.1, -90)
  line L80 (-115.1, -90) -> (-113.1, -90)
  line L81 (-113.1, -10) -> (-115.1, -10)
  line L82 (-113.1, -90) -> (-113.1, -10)
  line L83 (-120.1, -10) -> (-120.1, -90)
  line L84 (-120.1, -90) -> (-118.1, -90)
  line L85 (-118.1, -10) -> (-120.1, -10)
  line L86 (-118.1, -90) -> (-118.1, -10)
  line L87 (-125.1, -10) -> (-125.1, -90)
  line L88 (-125.1, -90) -> (-123.1, -90)
  line L89 (-123.1, -10) -> (-125.1, -10)
  line L90 (-123.1, -90) -> (-123.1, -10)
  point P0 (-74.1, -50)
  dimension "d332" = 2
  dimension "d333" = 80
  dimension "d336" = 5
  dimension "d337" = 0
  constraint midpoint L5 L8.start
  constraint midpoint L7 L8.end
  constraint horizontal L9
  constraint perpendicular L9 L10
  constraint parallel L9 L11
  constraint parallel L10 L12
  constraint coincident L13 P0
  constraint coincident L14 P0
  constraint midpoint L8 P0
  measures "d332" distance of L10.end L11.end
  measures "d333" distance of L9.end L10.end
extrude "Extrude26" cut sketch "bottom-cut-sketch" against normal blind 5 contours L9 L10 L11 L12 | L15 L16 L17 L18 | L19 L20 L21 L22 | L23 L24 L25 L26 | L27 L28 L29 L30 | L31 L32 L33 L34 | L35 L36 L37 L38 | L39 L40 L41 L42 | L43 L44 L45 L46 | L47 L48 L49 L50 | L51 L52 L53 L54 | L55 L56 L57 L58 | L59 L60 L61 L62 | L63 L64 L65 L66 | L67 L68 L69 L70 | L71 L72 L73 L74 | L75 L76 L77 L78 | L79 L80 L81 L82 | L83 L84 L85 L86 | L87 L88 L89 L90 bodies 1
named bodies: "case-bottom", "beetle-expansion", "main-case-body"
